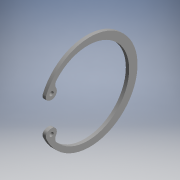
# Autodesk Inventor part: RRING-C-INT-S-55
Saved by Autodesk Inventor 2017.3 (Build 213256000, 256)
## iProperties
Part Number: RRING-C-INT-S-55
Material: Generic
Catalog Web Link: www.cadenas.de
Description: RRING_C_INT-Retaining Rings - C  (Internal)
Vendor: MISUMI
Document SubType Name: Modeling
Designer: partserver
Manufacturer: MISUMI
Mass: 1.27535 g
Surface Area: 19.3842 cm^2
Volume: 1.27535 cm^3
Density: 1 g/cm^3
Appearance: PSOLRGB-192-192-192
Category: PARTsolutions
Company: MISUMI
Title: RRING-C-INT-S-55
Author: Cadenas PARTsolutions
Comments: Retaining Rings - C  (Internal)
PSOL_IDENT_0: {$CADENAS_DATA\23d-libs\misumi\metric\accessories\rring_c_int.prj},181 {VTYP=3D},{NB=RRING-C-INT-S-5
PSOL_IDENT_1: 5},{LINA=RRING-C-INT-S-55},{NN=RRING_C_INT},{DATE=30.10.2020 15:47:10},{GEOMDATE=05.03.2015 00:00:00
PSOL_IDENT_2: },{VERSION=},{LINEID=250},{WBVAR=MAT},{WBNUMERIC=}  {NB=RRING-C-INT-S-55},{LINA=RRING-C-INT-S-55},{K
PSOL_IDENT_3: T=DUMMY},{PN=RRING-C-INT-S-55},{TYPE=RRING-C-INT},{MAT=-S},{HARD=36~44HRC},{NO=55},{DD3=59.2},{DD3TO
PSOL_IDENT_4: L=+0.45/-0.45},{TT=2.00},{TTTOL=+0.07/-0.07},{BB=5.1},{AA=6.5},{DD0=2.5},{DD4=41},{DD1=55},{DD2=58.0
PSOL_IDENT_5: },{DD2TOL=+0.3/0},{MM=2.20},{MMTOL=+0.14/0},{NN=2.0},{A2=21.50}
NB: RRING-C-INT-S-55
NN: 2
NT: Retaining Rings - C  (Internal)
NBSYN: $PN.
LINA: RRING-C-INT-S-55
CATALOG: Misumi
PN: RRING-C-INT-S-55
MAT: 304 Stainless Steel-CSP
HARD: 36~44HRC
NO: 55
DD3: 59.2
DD3TOL: +0.45/-0.45
TT: 2
TTTOL: +0.07/-0.07
BB: 5.1
AA: 6.5
DD0: 2.5
DD4: 41
DD1: 55
DD2: 58
DD2TOL: +0.3/0
MM: 2.2
MMTOL: +0.14/0
SUPPLIER: MISUMI
ARTICLENO: RRING-C-INT-S-55
BOMINFO: RRING-C-INT-S-55
CREATOR: CADENAS GmbH
Autodesk Inventor part; units mm, degrees
sketch "Sketch_3" plane through (0, 0, 0) normal (1, 0, 0) x (0, 1, 0)
  arc A0 (-26.7266, -11.2556) -> (-26.7266, 11.2556) centre (0, 0) ccw
  arc A1 (-26.7266, 11.2556) -> (-25.1712, 7.9) centre (-24.4226, 10.2853) ccw
  line L0 (-25.1712, 7.9) -> (-24.3719, 7.6491)
  arc A2 (-24.3719, 7.6491) -> (-20.6636, 12.5054) centre (-23.3987, 10.75) ccw
  arc A3 (-20.397, 16.3747) -> (-20.6636, 12.5054) centre (-17.9284, 14.2608) ccw
  arc A4 (-20.397, -16.3747) -> (-20.397, 16.3747) centre (-1.275, 0) ccw
  arc A5 (-20.6636, -12.5054) -> (-20.397, -16.3747) centre (-17.9284, -14.2608) ccw
  arc A6 (-20.6636, -12.5054) -> (-24.3719, -7.6491) centre (-23.3987, -10.75) ccw
  line L1 (-24.3719, -7.6491) -> (-25.1712, -7.9)
  arc A7 (-25.1712, -7.9) -> (-26.7266, -11.2556) centre (-24.4226, -10.2853) ccw
  circle A8 centre (-23.3987, -10.75) radius 1.25
  circle A9 centre (-23.3987, 10.75) radius 1.25
  constraints: 16 point on circle, 10 centre point, 4 end point
extrude "Extrusion1" add sketch "Sketch_3" along normal mid plane 2
ref_plane "rr_XY" through (-1, 0, 0) normal (1, 0, 0) x (0, 0, -1)
ref_plane "rr_YZ" through (-1, 0, 0) normal (0, 0, -1) x (0, 1, 0)
ref_plane "rr_ZX" through (-1, 0, 0) normal (0, 1, 0) x (1, 0, 0)
body "Solid1"
